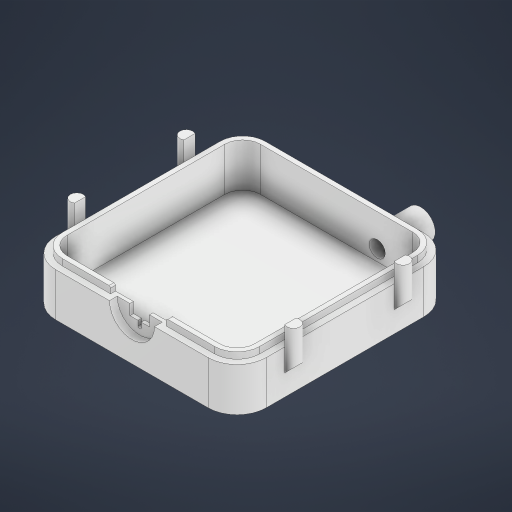
# Autodesk Inventor part: enclosure_down
Saved by Autodesk Inventor 2024 (Build 280153000, 153)
## iProperties
Created: 2023-07-19
Part Number: enclosure_down
Material: ABS Plastic
Document SubType Name: Modeling
Designer: LabTel_Admin
Density: 1.06 g/cm^3
Appearance: Smooth - White
Author: LabTel_Admin
Autodesk Inventor part; units mm, degrees
ref_plane "YZ Plane" through (0, 0, 0) normal (1, 0, 0) x (0, 1, 0)
ref_plane "XZ Plane" through (0, 0, 0) normal (0, 1, 0) x (-1, 0, 0)
sketch "Sketch1" plane through (0, 0, 0) normal (0, 1, 0) x (-1, 0, 0)
  line L0 (-23.65, -33.5) -> (23.65, -33.5)
  line L1 (32.65, -24.5) -> (32.65, 24.5)
  line L2 (23.65, 33.5) -> (-23.65, 33.5)
  line L3 (-32.65, 24.5) -> (-32.65, -24.5)
  line L4 (-32.65, -33.5) -> (32.65, 33.5) construction
  line L5 (32.65, -33.5) -> (-32.65, 33.5) construction
  arc A0 (32.65, 24.5) -> (23.65, 33.5) centre (23.65, 24.5) ccw
  arc A1 (23.65, -33.5) -> (32.65, -24.5) centre (23.65, -24.5) ccw
  arc A2 (-32.65, -24.5) -> (-23.65, -33.5) centre (-23.65, -24.5) ccw
  arc A3 (-23.65, 33.5) -> (-32.65, 24.5) centre (-23.65, 24.5) ccw
  line L6 (29.15, 24.5) -> (29.15, -24.5)
  arc A4 (23.65, -30) -> (29.15, -24.5) centre (23.65, -24.5) ccw
  line L7 (23.65, -30) -> (-23.65, -30)
  arc A5 (-29.15, -24.5) -> (-23.65, -30) centre (-23.65, -24.5) ccw
  line L8 (-29.15, -24.5) -> (-29.15, 24.5)
  arc A6 (-23.65, 30) -> (-29.15, 24.5) centre (-23.65, 24.5) ccw
  line L9 (-23.65, 30) -> (23.65, 30)
  arc A7 (29.15, 24.5) -> (23.65, 30) centre (23.65, 24.5) ccw
  point P0 (0, 0)
  point P1 (32.65, 0)
  point P2 (31.5, 26.5247)
  dimension "d3" = 9
  dimension "d4" = 9
  dimension "d5" = 3.5
  dimension "d75" = 58.3
  dimension "d76" = 60
  constraints: 20 end point, 16 point on circle, 8 centre point, 8 point on line, 8 tangent, 4 parallel, 3 midpoint, 2 equal radius, 2 perpendicular, 1 horizontal, 7 other
  measures "d3" radius of A0
  measures "d4" radius of A1
  measures "d5" distance between parallel lines of L1 L6
  measures "d75" distance between parallel lines of L8 L6
  measures "d76" distance between parallel lines of L9 L7
extrude "Extrusion1" add sketch "Sketch1" along normal blind 2 contours L6 A4 L7 A5 L8 A6 L9 A7
extrude "Extrusion2" add sketch "Sketch1" along normal blind 13.5
sketch "Sketch2" plane through (-23.65, 0, 33.5) normal (0, 0, 1) x (1, 0, 0)
  line L0 (0, 13.5) -> (47.3, 13.5) projected
  arc A0 (16.65, 13.5) -> (30.65, 13.5) centre (23.65, 13.5) ccw
  line L1 (16.65, 13.5) -> (30.65, 13.5)
  point P0 (23.65, 0)
  dimension "d10" = 14
  constraints: 2 end point, 2 point on circle, 2 point on line, 1 centre point, 1 collinear, 1 midpoint
  measures "d10" diameter of A0
extrude "Extrusion3" cut sketch "Sketch2" against normal blind 2.4
sketch "Sketch3" plane through (-23.65, 0, 31.1) normal (0, 0, 1) x (1, 0, 0)
  line L0 (26.7, 10.25) -> (20.6, 10.25)
  line L1 (20.6, 10.25) -> (20.6, 13.5)
  line L2 (26.7, 13.5) -> (26.7, 10.25)
  line L3 (16.65, 13.5) -> (30.65, 13.5) projected
  line L4 (26.7, 10.25) -> (23.65, 13.5) construction
  line L5 (20.6, 10.25) -> (26.7, 16.75) construction
  line L6 (20.6, 13.5) -> (26.7, 13.5)
  line L7 (24.15, 10.25) -> (24.15, 8.75)
  line L8 (23.65, 8.25) -> (23.65, 8.25)
  line L9 (23.15, 8.75) -> (23.15, 10.25)
  line L10 (23.65, 10.25) -> (24.15, 8.25) construction
  line L11 (23.65, 10.25) -> (23.15, 8.25) construction
  arc A0 (23.65, 8.25) -> (24.15, 8.75) centre (23.65, 8.75) ccw
  arc A1 (23.15, 8.75) -> (23.65, 8.25) centre (23.65, 8.75) ccw
  point P0 (23.65, 0)
  point P1 (23.65, 8.25)
  dimension "d13" = 6.5
  dimension "d15" = 1
  dimension "d17" = 0.5
  dimension "d91" = 6.1
  constraints: 22 end point, 8 point on line, 5 midpoint, 4 point on circle, 4 tangent, 2 centre point, 2 parallel, 1 concentric, 1 horizontal, 1 perpendicular
  measures "d13" distance of L5.end L0.start
  measures "d15" distance of L10.end L11.end
  measures "d17" radius of A0
  measures "d91" distance between parallel lines of L2 L1
extrude "Extrusion4" cut sketch "Sketch3" against normal blind 2
sketch "Sketch11" plane through (0, 13.5, 0) normal (0, 1, 0) x (1, 0, 0)
  line L0 (-32.65, 24.5) -> (-32.65, -24.5) projected
  line L1 (-32.65, 24.5) -> (-32.65, -24.5) projected
  arc A0 (-32.65, -24.5) -> (-23.65, -33.5) centre (-23.65, -24.5) ccw projected
  line L2 (-23.65, -33.5) -> (-7, -33.5) projected
  line L3 (7, -33.5) -> (23.65, -33.5) projected
  arc A1 (23.65, -33.5) -> (32.65, -24.5) centre (23.65, -24.5) ccw projected
  line L4 (32.65, -24.5) -> (32.65, 24.5) projected
  line L5 (32.65, -24.5) -> (32.65, 24.5) projected
  line L6 (32.65, -24.5) -> (32.65, 24.5) projected
  line L7 (23.65, 33.5) -> (-23.65, 33.5) projected
  line L8 (23.65, 33.5) -> (-23.65, 33.5) projected
  arc A2 (-23.65, 33.5) -> (-32.65, 24.5) centre (-23.65, 24.5) ccw projected
  line L9 (-32.65, 24.5) -> (-32.65, -24.5) projected
  line L10 (-29.15, 24.5) -> (-29.15, -24.5) projected
  line L11 (-30, 13) -> (-30, 13)
  line L12 (-30, -13) -> (-30, -13)
  line L13 (7, -31.1) -> (7, -33.5) projected
  line L14 (7, -30) -> (7, -31.1)
  line L15 (-7, -33.5) -> (-7, -31.1) projected
  line L16 (-23.65, -33.5) -> (23.65, -33.5) projected
  line L17 (8, -33.5) -> (23.65, -33.5)
  line L18 (32.65, -24.5) -> (32.65, 24.5)
  line L19 (23.65, 33.5) -> (-23.65, 33.5)
  line L20 (-32.65, 24.5) -> (-32.65, -24.5)
  line L21 (-23.65, -33.5) -> (-8.65, -33.5)
  arc A3 (-32.65, -24.5) -> (-23.65, -33.5) centre (-23.65, -24.5) ccw projected
  arc A4 (-32.65, -24.5) -> (-23.65, -33.5) centre (-23.65, -24.5) ccw
  arc A5 (-23.65, 33.5) -> (-32.65, 24.5) centre (-23.65, 24.5) ccw
  arc A6 (23.65, -33.5) -> (32.65, -24.5) centre (23.65, -24.5) ccw projected
  line L22 (-10.65, -31.5) -> (-10.65, -31.5)
  line L23 (-10.65, -31.5) -> (-23.65, -31.5)
  arc A7 (-30.65, -24.5) -> (-23.65, -31.5) centre (-23.65, -24.5) ccw
  line L24 (-30.65, -24.5) -> (-30.65, 24.5)
  arc A8 (-23.65, 31.5) -> (-30.65, 24.5) centre (-23.65, 24.5) ccw
  line L25 (-23.65, 31.5) -> (23.65, 31.5)
  line L26 (30.65, 21.5) -> (30.65, -24.4214)
  line L27 (-10.65, -31.5) -> (-8.65, -31.5)
  arc A9 (23.65, -33.5) -> (32.65, -24.5) centre (23.65, -24.5) ccw
  arc A10 (23.65, -31.5) -> (30.65, -24.5) centre (23.65, -24.5) ccw
  line L28 (23.65, -31.5) -> (23.5714, -31.5)
  line L29 (30.65, -24.5) -> (30.65, -24.4214)
  line L30 (23.65, -31.5) -> (8.65, -31.5)
  line L31 (8.65, -31.5) -> (8.65, -30)
  line L32 (-23.65, -30) -> (23.65, -30) projected
  line L33 (-8.65, -31.5) -> (-8.65, -30)
  line L34 (-8.65, -30) -> (-23.65, -30)
  arc A11 (-23.65, 30) -> (-29.15, 24.5) centre (-23.65, 24.5) ccw projected
  line L35 (-29.15, -24.5) -> (-29.15, 24.5)
  line L36 (23.65, 30) -> (-23.65, 30) projected
  line L37 (-23.65, 30) -> (23.65, 30)
  arc A12 (29.15, 24.5) -> (23.65, 30) centre (23.65, 24.5) ccw projected
  line L38 (29.15, 24.5) -> (29.15, -24.5)
  line L39 (23.65, -30) -> (8.65, -30)
  arc A13 (23.65, -30) -> (29.15, -24.5) centre (23.65, -24.5) ccw projected
  arc A14 (-23.65, 30) -> (-29.15, 24.5) centre (-23.65, 24.5) ccw
  arc A15 (29.15, 24.5) -> (23.65, 30) centre (23.65, 24.5) ccw
  arc A16 (32.65, 24.5) -> (23.65, 33.5) centre (23.65, 24.5) ccw projected
  arc A17 (32.65, 24.5) -> (23.65, 33.5) centre (23.65, 24.5) ccw
  arc A18 (23.65, -30) -> (29.15, -24.5) centre (23.65, -24.5) ccw
  arc A19 (-29.15, -24.5) -> (-23.65, -30) centre (-23.65, -24.5) ccw projected
  arc A20 (-29.15, -24.5) -> (-23.65, -30) centre (-23.65, -24.5) ccw
  line L40 (30.65, 21.5) -> (30.65, 24.5)
  arc A21 (30.65, 24.5) -> (23.65, 31.5) centre (23.65, 24.5) ccw
  point P0 (0, 0)
  point P1 (-32, 13)
  point P2 (-32, -13)
  point P3 (-32, -15)
  point P4 (-13, 32)
  point P5 (-15, 32)
  point P6 (-32, 15)
  point P7 (7, -32.3)
  dimension "d61" = 2
  dimension "d62" = 2
  constraints: 50 end point, 26 point on circle, 12 centre point, 8 tangent, 7 concentric, 6 horizontal, 4 point on line, 4 vertical, 3 collinear, 3 perpendicular, 2 parallel, 1 midpoint, 10 other
  measures "d62" radial gap between concentric circles of A1 A10
extrude "Extrusión11" add sketch "Sketch11" along normal blind 2 contours L10 A19 L32 L33 L27 L23 A7 L24 A8 L25 A21 L40 L26 L29 A10 L28 L30 L31 A13 L38 A12 L36 A11
fillet "Empalme2" radius 0.5 1 edges at (-8.65, 15.5, 30.75)
fillet "Empalme3" radius 0.5 1 edges at (8.65, 15.5, 30.75)
sketch "Boceto14" plane through (23.65, 0, -33.5) normal (0, 0, -1) x (-1, 0, 0)
  line L0 (-9, 0) -> (-9, 13.5) projected
  line L1 (0, 13.5) -> (47.3, 13.5) projected
  point P0 (23.65, 0)
  point P1 (11, 5.5)
  point P2 (-9, 13.4997)
  dimension "d82" = 20
  dimension "d83" = 8
  measures "d82" distance from line of L0 point (11, 5.5)
  measures "d83" distance from line of L1 point (11, 5.5)
hole "Agujero1" at (12.65, 5.5, -33.5) direction (0, 0, 1) diameter 5 depth 3.5
sketch "Boceto15" plane through (23.65, 0, -33.5) normal (0, 0, -1) x (-1, 0, 0)
  circle A0 centre (11, 5.5) radius 2.5 projected
  circle A1 centre (11, 5.5) radius 4.5
  circle A2 centre (11, 5.5) radius 2.5
  point P0 (23.65, 0)
  dimension "d92" = 9
  constraints: 2 centre point, 2 coincident, 1 concentric
  measures "d92" diameter of A1
extrude "Extrusión13" add sketch "Boceto15" along normal blind 10
fillet "Empalme8" radius 2 2 edges at (17.15, 5.5, -33.5) (15.15, 5.5, -43.5)
ref_plane "Plano de trabajo1" through (-36.65, 9.5, -13) normal (0, -1, 0) x (1, 0, 0)
sketch "Boceto16" plane through (-36.65, 9.5, -13) normal (0, -1, 0) x (1, 0, 0)
  line L0 (4, -11.5) -> (4, 37.5) projected
  line L1 (4, -6.5) -> (4, -1.5)
  circle A0 centre (3, -4) radius 2
  point P0 (36.65, 13)
  point P1 (4, -4)
  point P2 (4, -2.2679)
  point P3 (4, -5.7321)
  dimension "d96" = 5
  dimension "d97" = 5
  dimension "d99" = 1
  dimension "d100" = 4
  constraints: 2 coincident, 2 end point, 2 point on line, 1 centre point, 1 midpoint
  measures "d96" distance of L1.start L1.end
  measures "d97" distance of L1.start point (4, -11.5)
  measures "d99" distance of point (4, -4) point (3, -4)
  measures "d100" diameter of A0
extrude "Extrusión14" add sketch "Boceto16" against normal blind 10 contours A0 L0 picked at (2.492, -3.6342)
mirror "Simetría4" about plane through (0, 0, 0) normal (0, 0, 1) of "Extrusión14"
mirror "Simetría5" about plane through (0, 0, 0) normal (1, 0, 0) of "Extrusión14", "Simetría4"
chamfer "Chaflán3" distance 2.99 angle 45 4 edges at (-32.65, 9.5, 17) (32.65, 9.5, 17) (32.65, 9.5, -17) (-32.65, 9.5, -17)
body "Solid1"
